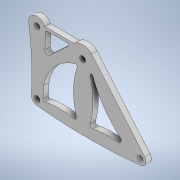
# Autodesk Inventor part: Bracket Concept MK11
Saved by Autodesk Inventor 2021 (Build 250183000, 183)
## iProperties
Created: 2021-05-11
Part Number: Bracket Concept MK11
Material: Generic
Document SubType Name: Modeling
Designer: Jawal
Density: 1 g/cm^3
Appearance: Default
Author: Jawal
Autodesk Inventor part; units mm, degrees
ref_plane "YZ Plane" through (0, 0, 0) normal (1, 0, 0) x (0, 1, 0)
ref_plane "XZ Plane" through (0, 0, 0) normal (0, 1, 0) x (-1, 0, 0)
ref_plane "XY Plane" through (0, 0, 0) normal (0, 0, 1) x (1, 0, 0)
sketch "Sketch1" plane through (0, 0, 0) normal (0, 0, 1) x (1, 0, 0)
  line L0 (-110, 70) -> (110, 70) construction
  line L1 (110, 70) -> (110, -70) construction
  line L2 (110, -70) -> (-110, -70) construction
  line L3 (-110, -70) -> (-110, 70) construction
  circle A0 centre (-90.0138, 55) radius 5
  circle A1 centre (-90.0214, -55) radius 5
  circle A2 centre (89.9786, -55) radius 5
  circle A3 centre (-10.4773, 45) radius 5
  line L4 (-67, 0) -> (-42, 0) construction
  line L5 (-42, 0) -> (-42, -30) construction
  line L6 (-42, -30) -> (-67, -30) construction
  line L7 (-67, -30) -> (-67, 0) construction
  circle A4 centre (-54.5, -19) radius 10 construction
  arc A5 (-76.3936, 61.2841) -> (-104.4102, 50.7876) centre (-90.0138, 55) ccw
  arc A6 (-99.9609, -53.9017) -> (-88.1312, -64.8197) centre (-90.0214, -55) ccw
  arc A7 (-100.0214, -55.005) -> (-105.0138, 54.9917) centre (-644.4166, -24.602) ccw
  line L8 (-35.5883, 51.8649) -> (-68.1439, 22.1865)
  line L9 (-75.3098, 53.8204) -> (-76.5077, 26.0974)
  line L10 (-78.8288, -29.0174) -> (-79.7785, -49.89)
  arc A8 (89.9786, -65) -> (97.6038, -48.5303) centre (89.9786, -55) ccw
  line L11 (4.9567, 60.6642) -> (97.6038, -48.5303)
  arc A9 (4.9567, 60.6642) -> (-25.2559, 61.2841) centre (-10.4773, 45) ccw
  arc A10 (-76.5077, 26.0974) -> (-68.1439, 22.1865) centre (-71.5124, 25.8816) ccw
  line L12 (-76.3936, 61.2841) -> (-25.2559, 61.2841)
  line L13 (-72.8121, 56.2124) -> (-37.2725, 56.2124)
  arc A11 (-72.8121, 56.2124) -> (-75.3098, 53.8204) centre (-72.8121, 53.7124) ccw
  arc A12 (-35.5883, 51.8649) -> (-37.2725, 56.2124) centre (-37.2725, 53.7124) ccw
  arc A13 (-20.0641, 28.3268) -> (-21.4793, -47.6907) centre (99.5505, -11.922) ccw
  circle A14 centre (-63.5274, -9.3914) radius 3 construction
  circle A15 centre (-57.919, -6.3914) radius 3 construction
  circle A16 centre (-51.0643, -6.3914) radius 3 construction
  circle A17 centre (-45.5038, -9.3914) radius 3 construction
  arc A18 (-23.0905, 31.5363) -> (-78.8288, -29.0174) centre (-2.761, -43.1063) ccw
  arc A19 (-20.0641, 28.3268) -> (-23.0905, 31.5363) centre (-22.4335, 29.1241) ccw
  arc A20 (-25.0801, -52.5035) -> (-21.4793, -47.6907) centre (-25.0756, -48.7535) ccw
  arc A21 (-79.7785, -49.89) -> (-77.2605, -52.5035) centre (-77.2811, -50.0036) ccw
  arc A22 (-90.0214, -65) -> (89.9786, -65) centre (-0.0214, 742.5) ccw
  arc A23 (-25.0801, -52.5035) -> (-77.2605, -52.5035) centre (-51.1703, -178.0833) ccw
  arc A24 (89.9786, -65) -> (97.6038, -48.5303) centre (89.9786, -55) ccw
  arc A25 (51.3169, -49.4442) -> (6.7008, -51.3162) centre (35.2009, -197.9611) ccw
  arc A26 (7.4915, 57.6767) -> (-25.2559, 61.2841) centre (-10.4773, 45) ccw
  arc A27 (2.5412, -46.1517) -> (6.7008, -51.3162) centre (5.9854, -47.6351) ccw
  arc A28 (51.3169, -49.4442) -> (55.6269, -41.1897) centre (51.8562, -44.4734) ccw
  arc A29 (2.5412, -46.1517) -> (2.5412, 27.2773) centre (-130.6751, -9.4372) ccw
  arc A30 (7.4934, 27.7888) -> (2.5825, 27.1273) centre (4.9934, 27.7888) ccw
  arc A31 (7.4934, 27.7888) -> (55.6269, -41.1897) centre (157.8186, 81.4032) ccw
  point P0 (0, 0)
  point P1 (-90.7944, -64.9701)
  point P2 (-90.0214, -65)
  dimension "d1" = 70
  dimension "d2" = 70
  dimension "d5" = 10
  dimension "d6" = 10
  dimension "d7" = 10
  dimension "d8" = 10
  dimension "d9" = 55
  dimension "d10" = 55
  dimension "d11" = 55
  dimension "d12" = 180
  dimension "d16" = 45
  dimension "d17" = 42
  dimension "d18" = 30
  dimension "d19" = 0
  dimension "d20" = 25
  dimension "d21" = 20
  dimension "d25" = 19
  dimension "d26" = 12.5
  dimension "d68" = 30
  dimension "d70" = 20
  dimension "d71" = 20
  dimension "d74" = 10
  dimension "d75" = 5
  dimension "d76" = 5
  dimension "d77" = 6
  dimension "d78" = 6
  dimension "d79" = 6
  dimension "d80" = 6
  dimension "d81" = 5
  dimension "d84" = 7.5
  dimension "d88" = 5
  dimension "d92" = 7.5
  dimension "d93" = 10
  dimension "d94" = 5
  constraints: 53 point on circle, 32 centre point, 28 end point, 18 tangent, 6 coincident, 5 parallel, 3 horizontal, 2 perpendicular, 1 point on line
  measures "d1" distance from line of point (0, 0) L2
  measures "d2" distance from line of point (0, 0) L0
  measures "d5" diameter of A0
  measures "d6" diameter of A1
  measures "d7" diameter of A2
  measures "d8" diameter of A3
  measures "d9" vertical distance of point (0, 0) A0.centre
  measures "d10" vertical distance of point (0, 0) A1.centre
  measures "d11" vertical distance of A2.centre point (0, 0)
  measures "d12" distance of A2.centre A1.centre
  measures "d16" vertical distance of point (0, 0) A3.centre
  measures "d17" distance from line of point (0, 0) L5
  measures "d18" distance of L4.end L5.end
  measures "d19" distance from line of L4 point (0, 0)
  measures "d20" distance of L5.end L6.end
  measures "d21" diameter of A4
  measures "d25" distance from line of L4 A4.centre
  measures "d26" distance from line of L7 A4.centre
  measures "d68" diameter of A5
  measures "d70" diameter of A6
  measures "d71" diameter of A8
  measures "d74" diameter of A10
  measures "d75" diameter of A11
  measures "d76" diameter of A12
  measures "d77" diameter of A14
  measures "d78" diameter of A15
  measures "d79" diameter of A16
  measures "d80" diameter of A17
  measures "d81" diameter of A19
  measures "d84" diameter of A20
  measures "d88" diameter of A21
  measures "d92" diameter of A27
  measures "d93" diameter of A28
  measures "d94" diameter of A30
extrude "Extrusion9" add sketch "Sketch1" along normal blind 9.4 contours L12 A9 L11 A8 A22 A6 A7 A5
equation "\"d1\" = d2"
equation "\"d10\" = d9"
equation "\"d11\" = d9"
equation "\"d26\" = 0.5 * d20"
body "Solid9"
